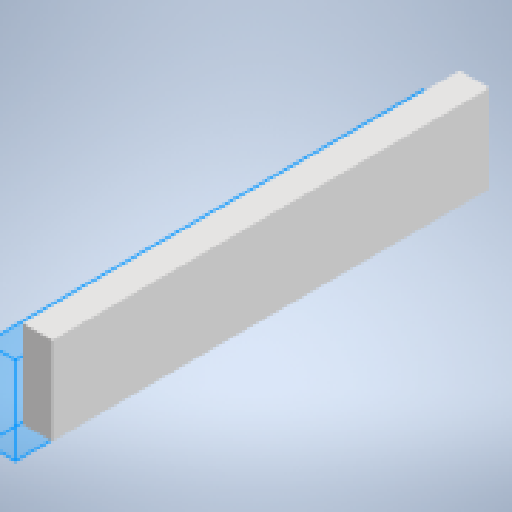
# Autodesk Inventor part: Part1
Saved by Autodesk Inventor 2025.3 (Build 293356000, 356)
## iProperties
Created: 2025-08-21
Part Number: Part1
Material: Steel
Document SubType Name: Modeling
Designer: steve
Mass: 576.975 g
Surface Area: 172.9 cm^2
Volume: 73.5 cm^3
Density: 7.85 g/cm^3
Appearance: Plate
Author: steve
Autodesk Inventor part; units mm, degrees
ref_plane "YZ Plane" through (0, 0, 0) normal (1, 0, 0) x (0, 1, 0)
ref_plane "XZ Plane" through (0, 0, 0) normal (0, 1, 0) x (-1, 0, 0)
ref_plane "XY Plane" through (0, 0, 0) normal (0, 0, 1) x (1, 0, 0)
sketch "Sketch1" plane through (0, 0, 0) normal (1, 0, 0) x (0, 1, 0)
  line L0 (-17.5, 87.5) -> (17.5, 87.5)
  line L1 (17.5, 87.5) -> (17.5, -87.5)
  line L2 (17.5, -87.5) -> (-17.5, -87.5)
  line L3 (-17.5, -87.5) -> (-17.5, 87.5)
  line L4 (-17.5, 87.5) -> (17.5, -87.5) construction
  line L5 (17.5, 87.5) -> (-17.5, -87.5) construction
  point P0 (0, 0)
  dimension "d0" = 35
  dimension "d1" = 175
  constraints: 12 end point, 2 midpoint, 2 parallel, 1 horizontal, 1 perpendicular
  measures "d0" distance between parallel lines of L3 L1
  measures "d1" distance between parallel lines of L0 L2
extrude "Extrusion1" add sketch "Sketch1" along normal blind 12
body "Solid1"
